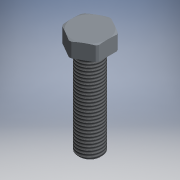
# Autodesk Inventor part: SLZ_63_Schraube_M16x60#
Saved by Autodesk Inventor 2017.3 (Build 213256000, 256)
## iProperties
Part Number: SLZ_63_Schraube_M16x60#
Material: Generic
Catalog Web Link: www.cadenas.de
Description: Schraube_SLZ 63-Control-Tec
Vendor: ROSEKRIEGER
Document SubType Name: Modeling
Designer: partserver
Manufacturer: ROSEKRIEGER
Mass: 17.3206 g
Surface Area: 47.9549 cm^2
Volume: 17.3206 cm^3
Density: 1 g/cm^3
Appearance: PSOLRGB-157-164-172
Category: PARTsolutions
Company: ROSEKRIEGER
Title: SLZ_63_Schraube_M16x60#
Author: Cadenas PARTsolutions
Comments: Control-Tec
PSOL_IDENT_0: {$CADENAS_DATA\23d-libs\rose_krieger\linearkomponenten\pool_lineartechnik\_hubsaeule_zyliinder\elekt
PSOL_IDENT_1: rozylinder\elekzyl_slz63\parts\slz63_plfl_schraube_16_60.prj},195 {VTYP=3D},{NB=SLZ_63_Schraube_M16x
PSOL_IDENT_2: 60#},{LINA=SLZ_63_Schraube_M16x60#},{NN=Schraube_SLZ 63},{DATE=02.12.2020 11:16:21},{GEOMDATE=22.06.
PSOL_IDENT_3: 2016 13:02:47},{VERSION=},{LINEID=10},{WBVAR=},{WBNUMERIC=}  {NB=SLZ_63_Schraube_M16x60#},{LINA=SLZ_
PSOL_IDENT_4: 63_Schraube_M16x60#},{KT=DUMMY},{IDNR=},{CODE=TQ3},{ARTIKEL=Elektrozylinder },{TYPE=SLZ 63 KG P PL},
PSOL_IDENT_5: {BEST=SLZ_63_Schraube_M16x60},{VARIANTE=PL},{SPINDEL=KG 25x10},{SPINDELCODE=3.000},{SCHUTZARTVIS=IP5
PSOL_IDENT_6: 4},{SCHUTZART=1},{HUB1=0,[0:100]},{HINWEINBAUX=Hub + 288,5 mm},{DUMMYDURCH=10.000},{DUMMYLAENG=20.00
PSOL_IDENT_7: 0},{HILFEHUB=105},{LAENDOPPROFIL=184.500},{RF=1.000},{GRUNDKOE=288.500},{A=100},{B=80},{C=100},{D=12
PSOL_IDENT_8: 5},{E=238},{F=40},{G=M16x1.5},{H=104},{K=125},{L=105},{M=48},{N=56.5},{O=86},{P=18.5},{PPATH=sbl_lz7
PSOL_IDENT_9: 0p_plfl.prj}
NB: SLZ_63_Schraube_M16x60#
NN: Schraube_SLZ 63
NT: Control-Tec
NBSYN: $BEST.#
LINA: SLZ_63_Schraube_M16x60#
CATALOG: RK Rose+Krieger
ARTIKEL: Elektrozylinder
TYPE: SLZ 63 KG P PL
BEST: SLZ_63_Schraube_M16x60
SPINDEL: KG 25x10
SPINDELCODE: 3
SCHUTZARTVIS: IP54
SCHUTZART: 1
HUB1: 0,[0:100]
HINWEINBAUX: Hub + 288,5 mm
HILFEHUB: 105
LAENDOPPROFIL: 184.5
GRUNDKOE: 288.5
A: 100
B: 80
C: 100
D: 125
E: 238
F: 40
G: M16x1.5
H: 104
K: 125
L: 105
M: 48
N: 56.5
O: 86
P: 18.5
SUPPLIER: ROSEKRIEGER
ARTICLENO: SLZ_63_Schraube_M16x60#
BOMINFO: SLZ_63_Schraube_M16x60#
CREATOR: CADENAS GmbH
Autodesk Inventor part; units mm, degrees
sketch "Sketch_3" plane through (0, 0, 0) normal (1, 0, 0) x (0, 0, -1)
  line L0 (10.8, 0) -> (-60, 0)
  line L1 (-60, 0) -> (-60, 6.773)
  line L2 (-60, 6.773) -> (-58.773, 8)
  line L3 (-58.773, 8) -> (-0.6, 8)
  arc A0 (-0.6, 8) -> (0, 8.6) centre (-0.6, 8.6) ccw
  line L4 (0, 8.6) -> (0, 11.25)
  line L5 (0, 11.25) -> (0.8, 11.7)
  line L6 (0.8, 11.7) -> (0.8, 13.38)
  line L7 (0.8, 13.38) -> (10.4302, 13.38)
  line L8 (10.4302, 13.38) -> (10.8, 12)
  line L9 (10.8, 12) -> (10.8, 0)
  line L10 (10.8, 0) -> (-60, 0)
  constraints: 22 end point, 2 point on circle, 1 centre point
revolve "Revolution1" add sketch "Sketch_3" angle 360 about axis through (0, 0, -10.8) along (0, 0, -1)
thread "Thread1" size "M16x2" class "6g" standard "ISO Metric profile" length 57.8748 offset 1.5252
sketch "Sketch_1" plane through (0, 0, 0) normal (0, 0, 1) x (1, 0, 0)
  line L0 (-24, -24) -> (24, -24)
  line L1 (24, -24) -> (24, 24)
  line L2 (24, 24) -> (-24, 24)
  line L3 (-24, 24) -> (-24, -24)
  line L4 (-12, -6.9282) -> (0, -13.8564)
  line L5 (0, -13.8564) -> (12, -6.9282)
  line L6 (12, -6.9282) -> (12, 6.9282)
  line L7 (12, 6.9282) -> (0, 13.8564)
  line L8 (0, 13.8564) -> (-12, 6.9282)
  line L9 (-12, 6.9282) -> (-12, -6.9282)
  constraints: 20 end point
extrude "Extrusion1" cut sketch "Sketch_1" against normal blind 10.8
ref_plane "DP402_XY" through (0, 6.773, 60) normal (1, 0, 0) x (0, 0, -1)
ref_plane "DP402_YZ" through (0, 6.773, 60) normal (0, 0, -1) x (0, 1, 0)
ref_plane "DP402_ZX" through (0, 6.773, 60) normal (0, 1, 0) x (1, 0, 0)
ref_plane "DPG1_XY" through (0, 8, 58.773) normal (1, 0, 0) x (0, 0, -1)
ref_plane "DPG1_YZ" through (0, 8, 58.773) normal (0, 0, -1) x (0, 1, 0)
ref_plane "DPG1_ZX" through (0, 8, 58.773) normal (0, 1, 0) x (1, 0, 0)
ref_plane "DPG2_XY" through (0, -8, 58.773) normal (1, 0, 0) x (0, 0, -1)
ref_plane "DPG2_YZ" through (0, -8, 58.773) normal (0, 0, -1) x (0, 1, 0)
ref_plane "DPG2_ZX" through (0, -8, 58.773) normal (0, 1, 0) x (1, 0, 0)
ref_plane "SCHRAUBE_XY" through (0, 0, 0) normal (0, 0, -1) x (1, 0, 0)
ref_plane "SCHRAUBE_YZ" through (0, 0, 0) normal (1, 0, 0) x (0, -1, 0)
ref_plane "SCHRAUBE_ZX" through (0, 0, 0) normal (0, -1, 0) x (0, 0, -1)
body "Solid1"
